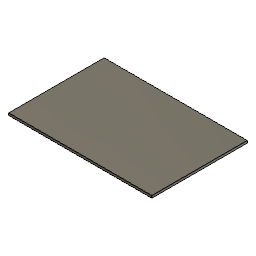
Top case (Autodesk Fusion 360 archive; units mm, degrees)
design "Top Cover"
part number: 2026-07-21-16-29-46-897
Autodesk Fusion 360 part; units mm, degrees
sketch "Sketch1" plane through (0, 0, 0) normal (0, 1, 0) x (1, 0, 0)
  line L0 (0, 0) -> (300, 0)
  line L1 (300, 0) -> (300, -200)
  line L2 (300, -200) -> (0, -200)
  line L3 (0, -200) -> (0, 0)
  dimension "d1" = 300
  dimension "d2" = 200
  constraint horizontal L0
  constraint vertical L1
  constraint horizontal L2
  constraint vertical L3
  constraint coincident L0.start L3.end
  measures "d1" distance of L0.start L0.end
  measures "d2" distance of L0.start L2.end
extrude "Extrude1" add sketch "Sketch1" along normal blind 5
